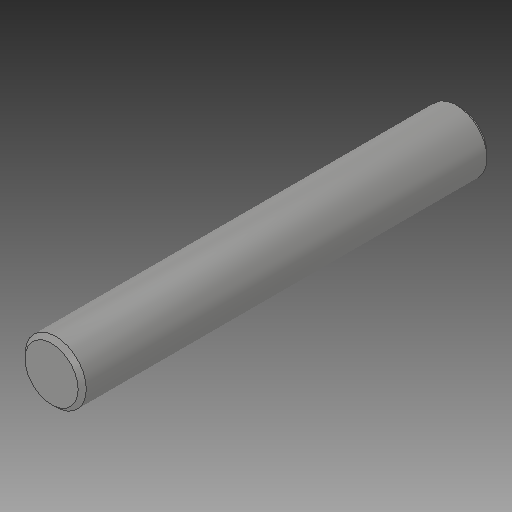
# Autodesk Inventor part: shaft_phi1.5_l6
Saved by Autodesk Inventor 2018.1 (Build 221171000, 171)
## iProperties
Part Number: shaft_phi1.5_l6
Material: 鋼
Document SubType Name: Modeling
Designer: sktom
Density: 7.85 g/cm^3
Appearance: プレート
Author: sktom
Autodesk Inventor part; units mm, degrees
ref_plane "YZ Plane" through (0, 0, 0) normal (1, 0, 0) x (0, 1, 0)
ref_plane "XZ Plane" through (0, 0, 0) normal (0, 1, 0) x (-1, 0, 0)
ref_plane "XY Plane" through (0, 0, 0) normal (0, 0, 1) x (1, 0, 0)
sketch "スケッチ1" plane through (0, 0, 0) normal (0, 0, 1) x (1, 0, 0)
  circle A0 centre (0, 0) radius 0.75
  dimension "d0" = 1.5
  constraints: 1 centre point, 1 coincident
  measures "d0" diameter of A0
extrude "押し出し1" add sketch "スケッチ1" along normal blind 10
chamfer "面取り1" distance 0.1 angle 45 2 edges at (-0.75, 0, 10) (-0.75, 0, 0)
